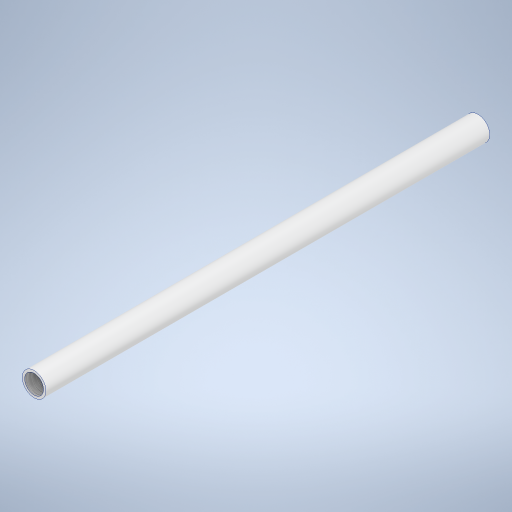
# Autodesk Inventor part: barra_Aluminio_8mm
Saved by Autodesk Inventor 2023 (Build 270158000, 158)
## iProperties
Created: 2023-07-16
Part Number: barra_Aluminio_8mm
Material: Aluminum 6061
Document SubType Name: Modeling
Designer: checo
Density: 2.7 g/cm^3
Appearance: Aluminum - Flat
units: mm
Author: checo
Autodesk Inventor part; units mm, degrees
ref_plane "YZ Plane" through (0, 0, 0) normal (1, 0, 0) x (0, 1, 0)
ref_plane "XZ Plane" through (0, 0, 0) normal (0, 1, 0) x (-1, 0, 0)
ref_plane "XY Plane" through (0, 0, 0) normal (0, 0, 1) x (1, 0, 0)
sketch "Sketch1" plane through (0, 0, 0) normal (0, 0, 1) x (1, 0, 0)
  circle A0 centre (0, 0) radius 4
  dimension "d0" = 8
  constraints: 1 centre point, 1 coincident
  measures "d0" diameter of A0
extrude "Extrusion1" add sketch "Sketch1" along normal blind 150
sketch "Sketch2" plane through (0, 0, 150) normal (0, 0, 1) x (1, 0, 0)
  point P0 (0, 0)
  point P1 (1.4516, 1.7573)
hole "Hole1" at (0, 0, 150) direction (0, 0, -1) diameter 6.35 depth 10 tip angle 118
thread "Thread1" size "1/4" designation "1/4 - 18 NPT" standard "NPT" length 15.103
body "Solid1"
